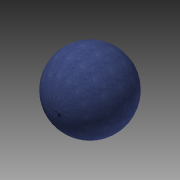
# Autodesk Inventor part: Ball
Saved by Autodesk Inventor 2013 (Build 170138000, 138)
## iProperties
Created: 2014-01-24
Part Number: Ball
Material: Generic
Document SubType Name: Modeling
Designer: Jarod
Density: 1 g/cm^3
Author: Jarod
Autodesk Inventor part; units mm, degrees
ref_plane "YZ Plane" through (0, 0, 0) normal (1, 0, 0) x (0, 1, 0)
ref_plane "XZ Plane" through (0, 0, 0) normal (0, 1, 0) x (-1, 0, 0)
ref_plane "XY Plane" through (0, 0, 0) normal (0, 0, 1) x (1, 0, 0)
sketch "Sketch1" plane through (0, 0, 0) normal (0, 1, 0) x (-1, 0, 0)
  circle A0 centre (0, 0) radius 304.8
  line L0 (301.5383, 44.4715) -> (-301.5383, -44.4715)
  dimension "d0" = 609.6
  constraints: 2 end point, 2 point on circle, 1 centre point, 1 coincident, 1 midpoint
  measures "d0" diameter of A0
revolve "Revolution1" add sketch "Sketch1" angle 360 about axis through (-301.5383, 0, 44.4715) along (0.9892988, 0, -0.1459038) picked at (58.0697, 109.5076) contours L0 A0
body "Solid1"
